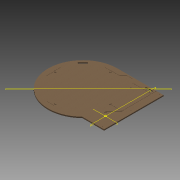
# Autodesk Inventor part: Base_Left
Saved by Autodesk Inventor 2014 SP1 (Build 180222100, 222)
## iProperties
Created: 2014-01-12
Part Number: Base_Left
Material: MDF Medium Density Fiberboard
Document SubType Name: Modeling
Designer: tuleu
Density: 0.8 g/cm^3
Appearance: Cardboard - Corrugated
Author: tuleu
Autodesk Inventor part; units mm, degrees
ref_plane "YZ Plane" through (0, 0, 0) normal (1, 0, 0) x (0, 1, 0)
ref_plane "XZ Plane" through (0, 0, 0) normal (0, 1, 0) x (-1, 0, 0)
ref_plane "XY Plane" through (0, 0, 0) normal (0, 0, 1) x (1, 0, 0)
sketch "Sketch1" plane through (0, 0, 0) normal (0, 1, 0) x (-1, 0, 0)
  arc A0 (0, -490) -> (-342.9286, 350) centre (0, 0) ccw
  line L0 (0, -490) -> (-650, -490)
  line L1 (-650, -490) -> (-650, 350)
  line L2 (-650, 350) -> (-342.9286, 350)
  dimension "d1" = 980
  dimension "d2" = 350
  dimension "d3" = 650
  constraints: 6 end point, 2 point on circle, 1 centre point, 1 coincident, 1 horizontal, 1 parallel, 1 perpendicular, 1 tangent
  measures "d1" diameter of A0
  measures "d2" distance from line of point (0, 0) L2
  measures "d3" distance from line of point (0, 0) L1
extrude "Extrusion1" add sketch "Sketch1" along normal mid plane 16
sketch "Sketch2" plane through (0, 8, 0) normal (0, 1, 0) x (1, 0, 0)
  arc A0 (0, 490) -> (342.9286, -350) centre (0, 0) ccw projected
  line L0 (650, -350) -> (650, 490) projected
  line L1 (650, 490) -> (0, 490) projected
  line L2 (435, 465) -> (525, 465)
  line L3 (530, 460) -> (530, 445)
  line L4 (525, 440) -> (435, 440)
  line L5 (430, 445) -> (430, 460)
  arc A1 (435, 465) -> (430, 460) centre (435, 460) ccw
  arc A2 (430, 445) -> (435, 440) centre (435, 445) ccw
  arc A3 (525, 440) -> (530, 445) centre (525, 445) ccw
  arc A4 (530, 460) -> (525, 465) centre (525, 460) ccw
  line L6 (0, 0) -> (-346.4823, 346.4823) construction
  line L7 (-289.9138, 353.5534) -> (-353.5534, 289.9138)
  line L8 (-353.5534, 282.8427) -> (-342.9468, 272.2361)
  line L9 (-335.8757, 272.2361) -> (-272.2361, 335.8757)
  line L10 (-272.2361, 342.9468) -> (-282.8427, 353.5534)
  arc A5 (-353.5534, 289.9138) -> (-353.5534, 282.8427) centre (-350.0179, 286.3782) ccw
  arc A6 (-342.9468, 272.2361) -> (-335.8757, 272.2361) centre (-339.4113, 275.7716) ccw
  arc A7 (-272.2361, 335.8757) -> (-272.2361, 342.9468) centre (-275.7716, 339.4113) ccw
  arc A8 (-282.8427, 353.5534) -> (-289.9138, 353.5534) centre (-286.3782, 350.0179) ccw
  point P0 (430, 465)
  point P1 (530, 465)
  point P2 (430, 440)
  dimension "d6" = 100
  dimension "d7" = 25
  dimension "d8" = 25
  dimension "d9" = 120
  dimension "d10" = 5
  dimension "d11" = 45
  dimension "d15" = 25
  dimension "d16" = 100
  dimension "d17" = 430
  dimension "d18" = 90
  dimension "d19" = 5
  constraints: 18 end point, 17 point on circle, 16 tangent, 8 centre point, 6 equal radius, 6 point on line, 4 parallel, 2 perpendicular, 1 horizontal, 1 other
  measures "d6" distance of point (430, 465) point (530, 465)
  measures "d7" distance of point (430, 440) point (430, 465)
  measures "d8" distance between parallel lines of L1 L2
  measures "d9" distance between parallel lines of L0 L3
  measures "d10" radius of A1
  measures "d11" angle of L0 L6
  measures "d15" distance between parallel lines of L9 L7
  measures "d16" distance between parallel lines of L8 L10
  measures "d17" distance from line of L6.start L9
  measures "d18" distance of L4.start L4.end
  measures "d19" radius of A5
extrude "Extrusion2" cut sketch "Sketch2" against normal through all
sketch "Sketch3" plane through (0, 8, 0) normal (0, 1, 0) x (1, 0, 0)
  circle A0 centre (610, 470) radius 4
  circle A1 centre (610, -330) radius 4
  circle A2 centre (610, 70) radius 4
  circle A3 centre (610, 470) radius 2.75 projected
  circle A4 centre (610, 70) radius 2.75 projected
  circle A5 centre (610, -330) radius 2.75 projected
  dimension "d22" = 8
  constraints: 3 centre point, 3 coincident, 2 equal radius
  measures "d22" diameter of A0
extrude "Extrusion3" cut sketch "Sketch3" against normal through all contours A0 | A1 | A2 | A3 | A4 | A5
ref_plane "Work Plane1" through (0, 0, 0) normal (-0.7071, 0, -0.7071) x (-0.7071, 0, 0.7071)
ref_plane "Work Plane2" through (500, 8, 350) normal (1, 0, 0) x (0, 0, -1)
ref_plane "Work Plane3" through (342.9286, 8, 180) normal (0, 0, 1) x (1, 0, 0)
sketch "Sketch5" plane through (0, 8, 0) normal (0, 1, 0) x (1, 0, 0)
  line L0 (530, 460) -> (530, 445) projected
  line L1 (525, 440) -> (435, 440) projected
  line L2 (-272.2361, 335.8757) -> (-335.8757, 272.2361) projected
  line L3 (650, 490) -> (0, 490) projected
  line L4 (570, 490) -> (570, -1.5)
  line L5 (570, -1.5) -> (565.3629, -1.5)
  line L6 (565.3629, -1.5) -> (444.4921, -122.3708)
  line L7 (75, 355) -> (-75, 355) construction
  line L8 (-75, 355) -> (-75, 205) construction
  line L9 (-75, 205) -> (75, 205) construction
  line L10 (75, 205) -> (75, 355) construction
  line L11 (197.9899, 304.0559) -> (304.0559, 197.9899) construction
  arc A0 (304.0559, 197.9899) -> (367.6955, 261.6295) centre (335.8757, 229.8097) ccw construction
  line L12 (367.6955, 261.6295) -> (261.6295, 367.6955) construction
  arc A1 (261.6295, 367.6955) -> (197.9899, 304.0559) centre (229.8097, 335.8757) ccw construction
  line L13 (-355, 75) -> (-355, -75) construction
  line L14 (-355, -75) -> (-205, -75) construction
  line L15 (-205, -75) -> (-205, 75) construction
  line L16 (-205, 75) -> (-355, 75) construction
  line L17 (355, -75) -> (355, 75) construction
  line L18 (355, 75) -> (205, 75) construction
  line L19 (205, 75) -> (205, -75) construction
  line L20 (205, -75) -> (355, -75) construction
  line L21 (-75, -355) -> (75, -355) construction
  line L22 (75, -355) -> (75, -205) construction
  line L23 (75, -205) -> (-75, -205) construction
  line L24 (-75, -205) -> (-75, -355) construction
  line L25 (485.8579, -229.4975) -> (549.4975, -165.8579) construction
  arc A2 (549.4975, -165.8579) -> (514.1421, -130.5025) centre (531.8198, -148.1802) ccw construction
  line L26 (514.1421, -130.5025) -> (450.5025, -194.1421) construction
  arc A3 (450.5025, -194.1421) -> (485.8579, -229.4975) centre (468.1802, -211.8198) ccw construction
  line L27 (205, 0) -> (355, 0) construction
  line L28 (0, 355) -> (0, 205) construction
  line L29 (251.0229, 251.0229) -> (314.6625, 314.6625) construction
  line L30 (-355, 0) -> (-205, 0) construction
  line L31 (0, -205) -> (0, -355) construction
  line L32 (482.3223, -162.3223) -> (517.6777, -197.6777) construction
  line L33 (550, 490) -> (550, 420)
  line L34 (550, 420) -> (284.2784, 420)
  line L35 (284.2784, 420) -> (234.2784, 470)
  line L36 (234.2784, 470) -> (148.6863, 470)
  line L37 (148.6863, 470) -> (96.6863, 418)
  line L38 (96.6863, 418) -> (-1.5, 418)
  line L39 (550, 409) -> (411.1213, 409)
  line L40 (411.1213, 409) -> (333.4008, 331.2795)
  line L41 (333.4008, 331.2795) -> (331.2795, 333.4008)
  line L42 (331.2795, 333.4008) -> (409.8787, 412)
  line L43 (280.9646, 412) -> (230.9646, 462)
  line L44 (230.9646, 462) -> (152, 462)
  line L45 (152, 462) -> (100, 410)
  line L46 (550, 409) -> (550, 1.5)
  line L47 (550, 1.5) -> (380, 1.5)
  line L48 (380, 1.5) -> (380, -1.5)
  line L49 (380, -1.5) -> (561.1203, -1.5)
  line L50 (561.1203, -1.5) -> (440.2495, -122.3708)
  line L51 (440.2495, -122.3708) -> (463.584, -145.7053)
  line L52 (463.584, -145.7053) -> (465.7053, -143.584)
  line L53 (465.7053, -143.584) -> (444.4921, -122.3708)
  line L54 (280.9646, 412) -> (409.8787, 412)
  line L55 (100, 410) -> (1.5, 410)
  line L56 (1.5, 410) -> (1.5, 380)
  line L57 (1.5, 380) -> (-1.5, 380)
  line L58 (-1.5, 380) -> (-1.5, 410)
  line L59 (-1.5, 410) -> (-100, 410)
  line L60 (-100, 410) -> (-410, 100)
  line L61 (-410, 100) -> (-410, 1.5)
  line L62 (-410, 1.5) -> (-380, 1.5)
  line L63 (-380, 1.5) -> (-380, -1.5)
  line L64 (-380, -1.5) -> (-410, -1.5)
  line L65 (-410, -1.5) -> (-410, -100)
  line L66 (-410, -100) -> (-100, -410)
  line L67 (-100, -410) -> (-1.5, -410)
  line L68 (-1.5, -410) -> (-1.5, -380)
  line L69 (-1.5, -380) -> (1.5, -380)
  line L70 (1.5, -380) -> (1.5, -413)
  line L71 (1.5, -413) -> (-101.2426, -413)
  line L72 (-101.2426, -413) -> (-413, -101.2426)
  line L73 (-413, -101.2426) -> (-413, -1.5)
  line L74 (-413, -1.5) -> (-416, -1.5)
  line L75 (-416, -1.5) -> (-416, 102.4853)
  line L76 (-416, 102.4853) -> (-102.4853, 416)
  line L77 (-102.4853, 416) -> (-1.5, 416)
  line L78 (-1.5, 416) -> (-1.5, 418)
  line L79 (550, 490) -> (570, 490)
  dimension "d33" = 25
  dimension "d34" = 3
  dimension "d35" = 3
  dimension "d36" = 3
  dimension "d37" = 55
  dimension "d38" = 25
  dimension "d39" = 20
  dimension "d40" = 20
  dimension "d41" = 20
  dimension "d42" = 11
  dimension "d43" = 3
  dimension "d44" = 25
  dimension "d45" = 45
  dimension "d46" = 8
  dimension "d47" = 8
  dimension "d48" = 20
  dimension "d49" = 8
  dimension "d50" = 25
  dimension "d51" = 3
  dimension "d52" = 55
  dimension "d53" = 6
  dimension "d54" = 8
  dimension "d55" = 8
  dimension "d56" = 25
  dimension "d57" = 6
  dimension "d58" = 25
  dimension "d59" = 3
  dimension "d60" = 55
  dimension "d61" = 6
  dimension "d62" = 25
  dimension "d63" = 3
  dimension "d64" = 3
  dimension "d65" = 25
  dimension "d66" = 3
  dimension "d67" = 25
  dimension "d68" = 3
  dimension "d69" = 55
  constraints: 112 end point, 37 parallel, 12 midpoint, 9 collinear, 8 perpendicular, 2 point on line, 1 vertical, 6 other
  measures "d33" distance between parallel lines of L52 L26
  measures "d34" distance between parallel lines of L51 L53
  measures "d35" distance between parallel lines of L50 L6
  measures "d36" distance between parallel lines of L5 L47
  measures "d37" distance between parallel lines of L26 L6
  measures "d38" distance between parallel lines of L48 L17
  measures "d39" distance between parallel lines of L33 L0
  measures "d40" distance between parallel lines of L4 L33
  measures "d41" distance between parallel lines of L34 L1
  measures "d42" distance between parallel lines of L39 L34
  measures "d43" distance between parallel lines of L40 L42
  measures "d44" distance between parallel lines of L41 L12
  measures "d45" distance between parallel lines of L12 L43
  measures "d46" distance between parallel lines of L44 L36
  measures "d47" distance between parallel lines of L43 L35
  measures "d48" distance between parallel lines of L3 L36
  measures "d49" distance between parallel lines of L34 L54
  measures "d50" distance between parallel lines of L7 L57
  measures "d51" distance between parallel lines of L56 L58
  measures "d52" distance between parallel lines of L7 L59
  measures "d53" distance between parallel lines of L59 L77
  measures "d54" distance between parallel lines of L55 L38
  measures "d55" distance between parallel lines of L45 L37
  measures "d56" distance from line of L45.end L10
  measures "d57" distance between parallel lines of L60 L76
  measures "d58" distance from line of L8 L59.end
  measures "d59" distance between parallel lines of L62 L64
  measures "d60" distance between parallel lines of L13 L61
  measures "d61" distance between parallel lines of L61 L75
  measures "d62" distance from line of L30.start L63
  measures "d63" distance between parallel lines of L65 L73
  measures "d64" distance between parallel lines of L70 L68
  measures "d65" distance between parallel lines of L21 L69
  measures "d66" distance between parallel lines of L71 L67
  measures "d67" horizontal distance of L21.start L66.end
  measures "d68" distance between parallel lines of L72 L66
  measures "d69" distance between parallel lines of L21 L67
extrude "Extrusion5" cut sketch "Sketch5" against normal blind 2.5
sketch "Sketch6" plane through (0, 8, 0) normal (0, 1, 0) x (1, 0, 0)
  line L0 (75, 355) -> (-75, 355) construction
  line L1 (-75, 355) -> (-75, 205) construction
  line L2 (-75, 205) -> (75, 205) construction
  line L3 (75, 205) -> (75, 355) construction
  line L4 (-355, 75) -> (-355, -75) construction
  line L5 (-355, -75) -> (-205, -75) construction
  line L6 (-205, -75) -> (-205, 75) construction
  line L7 (-205, 75) -> (-355, 75) construction
  line L8 (355, -75) -> (355, 75) construction
  line L9 (355, 75) -> (205, 75) construction
  line L10 (205, 75) -> (205, -75) construction
  line L11 (205, -75) -> (355, -75) construction
  line L12 (197.9899, 304.0559) -> (304.0559, 197.9899) construction
  arc A0 (304.0559, 197.9899) -> (367.6955, 261.6295) centre (335.8757, 229.8097) ccw construction
  line L13 (367.6955, 261.6295) -> (261.6295, 367.6955) construction
  arc A1 (261.6295, 367.6955) -> (197.9899, 304.0559) centre (229.8097, 335.8757) ccw construction
  line L14 (-75, -355) -> (75, -355) construction
  line L15 (75, -355) -> (75, -205) construction
  line L16 (75, -205) -> (-75, -205) construction
  line L17 (-75, -205) -> (-75, -355) construction
  line L18 (485.8579, -229.4975) -> (549.4975, -165.8579) construction
  arc A2 (549.4975, -165.8579) -> (514.1421, -130.5025) centre (531.8198, -148.1802) ccw construction
  line L19 (514.1421, -130.5025) -> (450.5025, -194.1421) construction
  arc A3 (450.5025, -194.1421) -> (485.8579, -229.4975) centre (468.1802, -211.8198) ccw construction
  line L20 (0, 355) -> (0, 205) construction
  line L21 (-355, 0) -> (-205, 0) construction
  line L22 (314.6625, 314.6625) -> (251.0229, 251.0229) construction
  line L23 (482.3223, -162.3223) -> (517.6777, -197.6777) construction
  line L24 (464.6447, -123.4315) -> (471.7157, -130.5025)
  line L25 (471.7157, -130.5025) -> (450.5025, -151.7157)
  line L26 (450.5025, -151.7157) -> (443.4315, -144.6447)
  line L27 (443.4315, -144.6447) -> (464.6447, -123.4315)
  line L28 (325.2691, 346.4823) -> (346.4823, 325.2691)
  line L29 (346.4823, 325.2691) -> (353.5534, 332.3402)
  line L30 (353.5534, 332.3402) -> (332.3402, 353.5534)
  line L31 (332.3402, 353.5534) -> (325.2691, 346.4823)
  line L32 (-15, 385) -> (15, 385)
  line L33 (15, 385) -> (15, 395)
  line L34 (15, 395) -> (-15, 395)
  line L35 (-15, 395) -> (-15, 385)
  line L36 (-395, 15) -> (-395, -15)
  line L37 (-395, -15) -> (-385, -15)
  line L38 (-385, -15) -> (-385, 15)
  line L39 (-385, 15) -> (-395, 15)
  line L40 (385, 15) -> (385, -15)
  line L41 (385, -15) -> (395, -15)
  line L42 (395, -15) -> (395, 15)
  line L43 (395, 15) -> (385, 15)
  line L44 (-15, -385) -> (15, -385)
  line L45 (15, -385) -> (15, -395)
  line L46 (15, -395) -> (-15, -395)
  line L47 (-15, -395) -> (-15, -385)
  dimension "d72" = 30
  dimension "d73" = 30
  dimension "d74" = 30
  dimension "d75" = 30
  dimension "d76" = 30
  dimension "d77" = 30
  dimension "d78" = 30
  dimension "d79" = 10
  constraints: 56 end point, 12 parallel, 10 equal length, 8 midpoint, 8 perpendicular, 6 other
  measures "d72" distance between parallel lines of L28 L13
  measures "d73" distance between parallel lines of L0 L32
  measures "d74" distance between parallel lines of L4 L38
  measures "d75" distance between parallel lines of L40 L8
  measures "d76" distance between parallel lines of L14 L44
  measures "d77" distance between parallel lines of L19 L25
  measures "d78" distance of L33.end L34.end
  measures "d79" distance between parallel lines of L32 L34
extrude "Extrusion6" cut sketch "Sketch6" against normal blind 6
body "Solid1"
